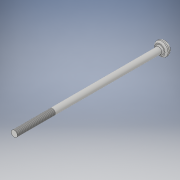
# Autodesk Inventor part: screw
Saved by Autodesk Inventor 2019 (Build 230136000, 136)
## iProperties
Created: 2021-01-19
Part Number: screw
Material: Generic
Document SubType Name: Modeling
Designer: CS
Density: 1 g/cm^3
Appearance: Default
Author: CS
Autodesk Inventor part; units mm, degrees
ref_plane "YZ Plane" through (0, 0, 0) normal (1, 0, 0) x (0, 1, 0)
ref_plane "XZ Plane" through (0, 0, 0) normal (0, 1, 0) x (-1, 0, 0)
ref_plane "XY Plane" through (0, 0, 0) normal (0, 0, 1) x (1, 0, 0)
sketch "Sketch1" plane through (0, 0, 0) normal (0, 0, 1) x (1, 0, 0)
  circle A0 centre (0, 0) radius 0.4
  circle A1 centre (0, 0) radius 0.875
  dimension "d0" = 0.8
  dimension "d1" = 1.75
  constraints: 2 centre point, 2 coincident
  measures "d0" diameter of A0
  measures "d1" diameter of A1
extrude "Extrusion1" add sketch "Sketch1" along normal blind 19 contours A0
extrude "Extrusion2" add sketch "Sketch1" against normal blind 0.75 contours A0 | A1
thread "Thread1" size "M0.8x0.2" class "6g" standard "ANSI Metric M Profile" length 5
fillet "Fillet1" radius 0.4 1 edges at (-0.875, 0, -0.75)
fillet "Fillet2" radius 0.2 1 edges at (-0.875, 0, 0)
fillet "Fillet3" radius 0.15 1 edges at (-0.4, 0, 0)
sketch "Sketch2" plane through (0, 0, -0.75) normal (0, 0, -1) x (-1, 0, 0)
  line L0 (-0.75, 0.3) -> (0.75, 0.3)
  line L1 (0.75, 0.3) -> (0.75, -0.3)
  line L2 (0.75, -0.3) -> (-0.75, -0.3)
  line L3 (-0.75, -0.3) -> (-0.75, 0.3)
  line L4 (-0.3, 0.75) -> (0.3, 0.75)
  line L5 (0.3, 0.75) -> (0.3, -0.75)
  line L6 (0.3, -0.75) -> (-0.3, -0.75)
  line L7 (-0.3, -0.75) -> (-0.3, 0.75)
  point P0 (0, 0)
  point P1 (0, 0.3)
  point P2 (0, 0.75)
  point P3 (-0.75, 0)
  point P4 (-0.3, 0)
  dimension "d11" = 1.5
  dimension "d12" = 0.6
  constraints: 16 end point, 4 midpoint, 4 parallel, 4 perpendicular, 2 horizontal, 2 horizontal alignment, 2 vertical alignment
  measures "d11" distance between parallel lines of L6 L4
  measures "d12" distance of L4.start L4.end
sketch "Sketch3" plane through (0, 0, 0) normal (0, 0, 1) x (1, 0, 0)
  circle A0 centre (0, 0) radius 0.375
  dimension "d13" = 0.75
  constraints: 1 centre point, 1 coincident
  measures "d13" diameter of A0
loft "Loft1" cut profiles "Sketch2", "Sketch3"
fillet "Fillet4" radius 0.15 4 edges at (0.2826, 0.2826, -0.375) (-0.2826, 0.2826, -0.375) (0.2826, -0.2826, -0.375) (-0.2826, -0.2826, -0.375)
body "Solid1"
